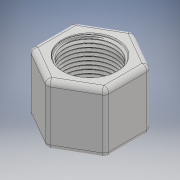
# Autodesk Inventor part: Acople
Saved by Autodesk Inventor 2018.3 (Build 223284000, 284)
## iProperties
Created: 2020-02-26
Part Number: Acople
Material: Generic
Document SubType Name: Modeling
Designer: Ivan
Density: 1 g/cm^3
Appearance: Default
Author: Ivan
Autodesk Inventor part; units mm, degrees
ref_plane "YZ Plane" through (0, 0, 0) normal (1, 0, 0) x (0, 1, 0)
sketch "Sketch14" plane through (0, 0, 0) normal (0, 0, 1) x (1, 0, 0)
  circle A0 centre (0, 0) radius 11
  circle A1 centre (0, 0) radius 17.5
  dimension "d66" = 22
  dimension "d67" = 35
  constraints: 2 centre point, 2 coincident
  measures "d66" diameter of A0
  measures "d67" diameter of A1
extrude "Extrusion4" add sketch "Sketch14" along normal blind 24
thread "Thread2" size "M22x1.5" class "6H" standard "ANSI Metric M Profile" full length
sketch "Sketch16" plane through (0, 0, 24) normal (-1, 0, 0) x (0, 1, 0)
  line L0 (11, 0) -> (11, 24)
  line L1 (11, 24) -> (9.8878, 24)
  line L2 (9.8878, 24) -> (9.8878, 0)
  line L3 (9.8878, 0) -> (11, 0)
  line L4 (0, -4.8) -> (0, 28.8) projected
  constraints: 8 end point
revolve "Revolution2" add sketch "Sketch16" angle 360 about axis through (0, 0, 24) along (0, 0, -1) separate body
sketch "Sketch15" plane through (0, 11, 24) normal (1, 0, 0) x (0, 0, -1)
  line L0 (-0.8751, -0.076) -> (-0.7501, -0.076) construction
  line L1 (0.1249, -1.0365) -> (-0.0001, -1.2766) construction
  line L2 (-1.5001, -1.2766) -> (-1.6251, -1.0365) construction
  line L3 (-0.6251, -0.076) -> (-0.7501, 0.1641) construction
  line L4 (-0.7501, 0.1641) -> (-0.8751, -0.076) construction
  line L5 (-1.5001, -1.2766) -> (-1.3751, -1.0365) construction
  line L6 (-0.6251, -0.076) -> (-0.1251, -1.0365)
  line L7 (-1.6251, -1.0365) -> (-1.3751, -1.0365) construction
  arc A0 (-1.6251, -1.0365) -> (-1.5001, -1.1124) centre (-1.5001, -0.9714) ccw construction
  line L8 (0.1249, -1.0365) -> (-0.1251, -1.0365) construction
  line L9 (-1.5001, -1.2766) -> (-1.5001, -1.0365) construction
  line L10 (-0.0001, -1.2766) -> (-0.0001, -1.0365) construction
  line L11 (-0.7501, 0.1641) -> (-0.7501, -0.0002) construction
  line L12 (-1.5001, -1.1124) -> (-0.0001, -1.1124)
  arc A1 (-1.5001, -1.1124) -> (-1.3751, -1.0365) centre (-1.5001, -0.9714) ccw
  line L13 (-0.1251, -1.0365) -> (-0.0001, -1.2766) construction
  line L14 (-1.3751, -1.0365) -> (-0.8751, -0.076)
  line L15 (-0.0001, -0.0002) -> (-0.0001, 0.0177)
  line L16 (-0.0001, 0.0177) -> (-0.0001, -0.0002)
  line L17 (-0.0001, -0.0002) -> (0.0334, -0.0002)
  arc A2 (-0.1251, -1.0365) -> (-0.0001, -1.1124) centre (-0.0001, -0.9714) ccw
  arc A3 (-0.0001, -1.1124) -> (0.1249, -1.0365) centre (-0.0001, -0.9714) ccw construction
  arc A4 (-0.7501, -0.0002) -> (-0.8751, -0.076) centre (-0.7501, -0.1411) ccw
  arc A5 (-0.6251, -0.076) -> (-0.7501, -0.0002) centre (-0.7501, -0.1411) ccw
  line L18 (-0.7501, -0.0002) -> (-0.7501, -0.076) construction
  line L19 (-0.7501, -0.076) -> (-0.6251, -0.076) construction
  dimension "d72" = 55
  dimension "d73" = 0.2401
  dimension "d74" = 0.2401
  dimension "Sketch15_ThreadOffset" = 0
  dimension "Sketch15_MajorRadius" = 1.1122
  dimension "d77" = 1.5
  dimension "Sketch15_MinorRadius" = 0
  constraints: 40 end point, 12 point on circle, 10 parallel, 8 tangent, 6 centre point, 6 collinear, 2 midpoint, 2 point on line, 1 horizontal, 1 perpendicular, 3 other
  measures "d72" angle of L6 L14
  measures "d73" distance of L3.end L0.end
  measures "d74" distance of L1.end L10.end
  measures "Sketch15_ThreadOffset" distance between parallel lines of L15 L10
  measures "Sketch15_MajorRadius" distance from line of L12 L15.start
  measures "d77" distance from line of L1.end L9
  measures "Sketch15_MinorRadius" distance edge to line of A5 L17
coil "Coil2" sketch "Sketch15" operation cut axis through (0, 0, 24) along (0, 0, -1) pitch 1.5015 turns 17.982018 hand right bodies 2
ref_plane "Work Plane5" through (0, 0, 23) normal (0, 0, 1) x (1, 0, 0)
sketch "Sketch17" plane through (0, 0, 23) normal (0, 0, 1) x (1, 0, 0)
  circle A0 centre (0, 0) radius 10.5
  dimension "d91" = 21
  constraints: 1 centre point, 1 coincident
  measures "d91" diameter of A0
sketch "Sketch18" plane through (0, 0, 24) normal (0, 0, 1) x (1, 0, 0)
  circle A0 centre (0, 0) radius 11
  dimension "d92" = 22
  constraints: 1 centre point, 1 coincident
  measures "d92" diameter of A0
loft "Loft6" cut profiles "Sketch18", "Sketch17" bodies 1 2
ref_plane "Work Plane6" through (0, 0, 12) normal (0, 0, 1) x (1, 0, 0)
mirror "Mirror1" about plane through (0, 0, 12) normal (0, 0, 1) of "Loft6" bodies 1 2
sketch "Sketch19" plane through (0, 0, 24) normal (0, 0, 1) x (1, 0, 0)
  circle A0 centre (0, 0) radius 17.5 projected
  line L0 (0, 17.5) -> (15.1554, 8.75)
  line L1 (15.1554, 8.75) -> (15.1554, -8.75)
  line L2 (15.1554, -8.75) -> (0, -17.5)
  line L3 (0, -17.5) -> (-15.1554, -8.75)
  line L4 (-15.1554, -8.75) -> (-15.1554, 8.75)
  line L5 (-15.1554, 8.75) -> (0, 17.5)
  constraints: 12 end point, 1 coincident, 1 vertical alignment, 14 other
extrude "Extrusion5" cut sketch "Sketch19" against normal blind 24 contours A0 L1 | L0 A0 | A0 L2 | L5 A0 | A0 L3 | L4 A0 bodies 1
fillet "Fillet5" radius 2 12 edges at (7.5777, 13.125, 24) (-7.5777, 13.125, 24) (-15.1554, 0, 24) (-7.5777, -13.125, 24) (7.5777, -13.125, 24) (15.1554, 0, 24) (7.5777, 13.125, 0) (-7.5777, 13.125, 0) (-15.1554, 0, 0) (-7.5777, -13.125, 0) (7.5777, -13.125, 0) (15.1554, 0, 0)
fillet "Fillet6" radius 2 18 edges at (0, 16.8236, 23.4142) (0, 16.8236, 0.5858) (0, 17.5, 12) (14.5697, 8.4118, 0.5858) (14.5697, 8.4118, 23.4142) (15.1554, 8.75, 12) (14.5697, -8.4118, 0.5858) (14.5697, -8.4118, 23.4142) (15.1554, -8.75, 12) (0, -16.8236, 0.5858) (0, -16.8236, 23.4142) (0, -17.5, 12) (-14.5697, -8.4118, 0.5858) (-14.5697, -8.4118, 23.4142) (-15.1554, -8.75, 12) (-14.5697, 8.4118, 0.5858) (-14.5697, 8.4118, 23.4142) (-15.1554, 8.75, 12)
equation "\"d72\" = d79"
equation "\"d73\" = 0.160083 * Sketch15_Pitch"
equation "\"d74\" = 0.160083 * Sketch15_Pitch"
equation "\"d77\" = Sketch15_Pitch"
equation "\"d30\" = 55deg"
equation "\"Sketch7_Pitch\" = 1.5"
equation "\"d79\" = 55deg"
equation "\"Sketch15_Pitch\" = 1.5"
body "Solid3"
body "Solid4"
